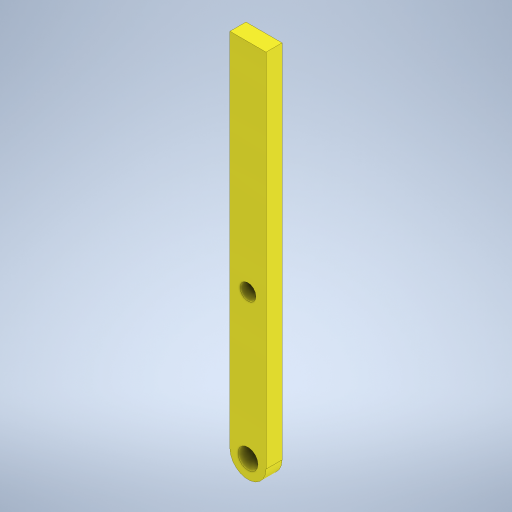
# Autodesk Inventor part: 1-HUDSON-8-33-TDR HAND PUMP HANDLE
Saved by Autodesk Inventor 2024.2 (Build 282272000, 272)
## iProperties
Created: 2024-11-01
Part Number: 1-HUDSON-8-33-TDR HAND PUMP HANDLE
Material: Genérico
Document SubType Name: Modeling
Designer: brene
Density: 1 g/cm^3
Appearance: Canario
Author: brene
Autodesk Inventor part; units mm, degrees
ref_plane "YZ Plane" through (0, 0, 0) normal (1, 0, 0) x (0, 1, 0)
ref_plane "XZ Plane" through (0, 0, 0) normal (0, 1, 0) x (-1, 0, 0)
ref_plane "XY Plane" through (0, 0, 0) normal (0, 0, 1) x (1, 0, 0)
sketch "Boceto1" plane through (0, 0, 0) normal (0, 0, 1) x (1, 0, 0)
  line L0 (0, 55.8594) -> (0, -55.8594) construction
  line L1 (110.1563, 0) -> (-110.1563, 0) construction
  line L2 (-4.5, 41.4844) -> (4.5, 41.4844)
  line L3 (4.5, 41.4844) -> (4.5, -48.5156)
  line L4 (4.5, -48.5156) -> (-4.5, -48.5156)
  line L5 (-4.5, -48.5156) -> (-4.5, 41.4844)
  arc A0 (-4.5, -48.5156) -> (4.5, -48.5156) centre (0, -48.5156) ccw
  circle A1 centre (0, -48.5156) radius 2.5
  point P0 (0, 0)
  point P1 (0, 0)
  point P2 (0, 41.4844)
  point P3 (0, -12.5156)
  point P4 (0, -48.5156)
  dimension "d0" = 90
  dimension "d1" = 9
  dimension "d2" = 4.5
  dimension "d3" = 5
  dimension "d4" = 36
  dimension "d5" = 41.4844
  dimension "d6" = 105.6563
  dimension "d7" = 55.8594
  constraints: 12 end point, 4 midpoint, 2 centre point, 2 coincident, 2 horizontal, 2 parallel, 2 point on circle, 2 point on line, 2 tangent, 1 perpendicular, 1 vertical
  measures "d0" distance of L2.end L3.end
  measures "d1" distance of L2.start L2.end
  measures "d2" radius of A0
  measures "d3" diameter of A1
  measures "d4" distance of point (0, -12.516) point (0, -48.516)
  measures "d5" distance between parallel lines of L1 L2
  measures "d6" distance from line of L1.start L3
  measures "d7" distance from line of L0.start L1
extrude "Extrusión1" add sketch "Boceto1" against normal blind 4 contours L2 L3 L4 A1 L5 | L4 A1 A0
hole "Agujero1" at (0, -12.5156, 0) direction (0, 0, -1) diameter 4 end through all
